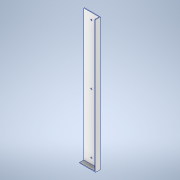
# Autodesk Inventor part: Guias de bandeja 1
Saved by Autodesk Inventor 2020 (Build 240168000, 168)
## iProperties
Created: 2020-05-08
Part Number: Guias de bandeja 1
Material: Aluminio 6061
Document SubType Name: Modeling
Designer: Pipi
Density: 2.7 g/cm^3
Appearance: Aluminio - Plano
Author: Pipi
Autodesk Inventor part; units mm, degrees
ref_plane "YZ Plane" through (0, 0, 0) normal (1, 0, 0) x (0, 1, 0)
ref_plane "XZ Plane" through (0, 0, 0) normal (0, 1, 0) x (-1, 0, 0)
ref_plane "XY Plane" through (0, 0, 0) normal (0, 0, 1) x (1, 0, 0)
sketch "Boceto1" plane through (0, 0, 0) normal (0, 1, 0) x (-1, 0, 0)
  line L0 (40.8526, 17.8417) -> (40.8526, 15.8417)
  line L1 (40.8526, 15.8417) -> (-9.1474, 15.8417)
  line L2 (-9.1474, 15.8417) -> (-9.1474, 30.8417)
  line L3 (-9.1474, 30.8417) -> (-7.1474, 30.8417)
  line L4 (-7.1474, 30.8417) -> (-7.1474, 17.8417)
  line L5 (-7.1474, 17.8417) -> (40.8526, 17.8417)
  dimension "d0" = 2
  dimension "d1" = 50
  dimension "d2" = 15
  dimension "d3" = 2
  constraints: 12 end point, 5 perpendicular, 1 vertical
  measures "d0" distance of L0.start L0.end
  measures "d1" distance of L0.end L1.end
  measures "d2" distance of L1.end L2.end
  measures "d3" distance of L2.end L3.end
extrude "Extrusión1" add sketch "Boceto1" along normal blind 414
sketch "Boceto3" plane through (-40.8526, 0, 17.8417) normal (0, 0, 1) x (1, 0, 0)
  line L0 (0, 0) -> (48, 0) projected
  line L1 (0, 414) -> (48, 414) projected
  line L2 (0, 0) -> (0, 414) projected
  line L3 (0, 207) -> (48, 207)
  line L4 (48, 0) -> (48, 414) projected
  line L5 (48, 0) -> (50, 0) projected
  line L6 (48, 0) -> (24, 0)
  line L7 (24, 0) -> (24, 414)
  circle A0 centre (24, 207) radius 2
  line L8 (24, 0) -> (24, 20)
  line L9 (24, 414) -> (24, 394)
  circle A1 centre (24, 20) radius 2
  circle A2 centre (24, 394) radius 2
  point P0 (40.8526, 0)
  dimension "d8" = 24
  dimension "d9" = 414
  dimension "d10" = 4
  dimension "d11" = 20
  dimension "d13" = 4
  dimension "d14" = 4
  constraints: 10 end point, 5 midpoint, 3 centre point, 2 coincident, 2 point on line
  measures "d8" distance of L0.end L6.end
  measures "d9" distance of L6.end L7.end
  measures "d10" diameter of A0
  measures "d11" distance of L6.end L8.end
  measures "d13" diameter of A1
  measures "d14" diameter of A2
extrude "Extrusión2" cut sketch "Boceto3" against normal blind 10 contours A1 L7 | L7 A1 | A0 L7 L3 | L3 L7 A0 | L7 A0 L3 | L3 A0 L7 | A2 L7 | L7 A2
sketch "Boceto4" plane through (-40.8526, 0, 17.8417) normal (0, 0, 1) x (1, 0, 0)
  line L0 (50, 0) -> (0, 0) projected
  line L1 (0, 0) -> (0, 2)
  line L2 (0, 2) -> (48, 2)
  line L3 (48, 0) -> (48, 414) projected
  line L4 (48, 2) -> (48, 0)
  line L5 (48, 0) -> (0, 0)
  point P0 (40.8526, 0)
  dimension "d17" = 2
  constraints: 8 end point, 2 vertical, 1 parallel, 1 perpendicular, 1 point on line
  measures "d17" distance of L0.end L1.end
extrude "Extrusión3" add sketch "Boceto4" along normal blind 13
